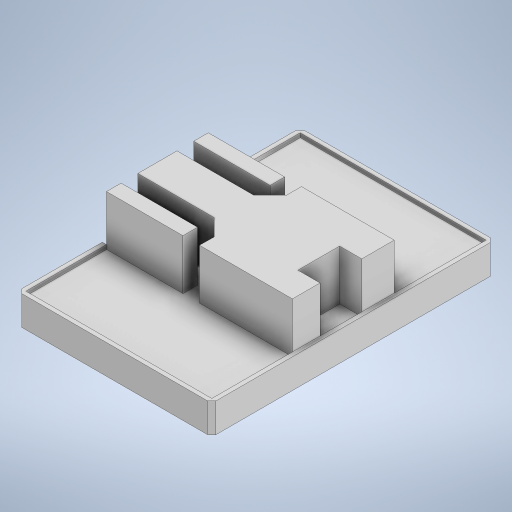
# Autodesk Inventor part: Suporte
Saved by Autodesk Inventor 2024 (Build 280153020, 153B)
## iProperties
Created: 2023-05-31
Part Number: Suporte
Material: Genérico
Document SubType Name: Modeling
Designer: victo
Density: 1 g/cm^3
Appearance: Padrão
Author: victo
Autodesk Inventor part; units mm, degrees
ref_plane "YZ Plane" through (0, 0, 0) normal (1, 0, 0) x (0, 1, 0)
ref_plane "XZ Plane" through (0, 0, 0) normal (0, 1, 0) x (-1, 0, 0)
ref_plane "XY Plane" through (0, 0, 0) normal (0, 0, 1) x (1, 0, 0)
sketch "Esboço1" plane through (0, 0, 0) normal (0, 1, 0) x (-1, 0, 0)
  line L0 (0.0003, 60.0007) -> (0.0003, 29.9998)
  line L1 (0.0003, 29.9998) -> (0.0003, 29.9999)
  line L2 (-0.9997, 29.9999) -> (-0.9997, 60.0007)
  line L3 (0.0003, 29.9999) -> (0.0003, 14.4635)
  line L4 (-0.9997, 14.4635) -> (-0.9997, 29.9999)
  line L5 (44.5003, 33.7635) -> (45.5003, 33.7635)
  line L6 (44.5003, 58.1254) -> (45.5003, 58.1254)
  line L7 (26.2003, 33.7635) -> (26.2003, 37.2635)
  line L8 (26.2003, 37.2635) -> (44.5003, 37.2635)
  line L9 (22.2003, 33.7635) -> (0.0003, 33.7635)
  line L10 (22.2003, 33.7635) -> (22.2003, 37.2635)
  line L11 (26.2003, 33.7635) -> (45.0003, 33.7635)
  line L12 (37.268, 41.2635) -> (44.5003, 41.2635)
  line L13 (22.2003, 37.2635) -> (26.2003, 41.2635)
  line L14 (37.268, 41.2635) -> (26.2003, 41.2635)
  line L15 (43.0622, 54.6254) -> (44.5003, 54.6254)
  line L16 (43.0622, 54.6254) -> (26.2003, 54.6254)
  line L17 (26.2003, 54.6254) -> (26.2003, 58.1254)
  line L18 (22.2003, 54.6254) -> (22.2503, 58.1254)
  line L19 (26.2003, 50.6254) -> (22.2003, 54.6254)
  line L20 (26.2003, 50.6254) -> (44.5003, 50.6254)
  line L21 (0.0003, 58.1254) -> (22.2503, 58.1254)
  line L22 (26.2003, 58.1254) -> (44.5003, 58.1254)
  line L23 (44.5003, 54.6254) -> (44.5003, 58.1254)
  line L24 (44.5003, 48.0257) -> (44.5003, 50.6254)
  line L25 (44.5003, 33.7635) -> (44.5003, 37.2635)
  line L26 (44.5003, 41.2635) -> (44.5003, 45.0257)
  line L27 (44.5003, 37.2635) -> (44.5003, 41.2635)
  line L28 (44.5003, 45.0257) -> (44.5003, 48.0257)
  line L29 (44.5003, 50.6254) -> (44.5003, 54.6254)
  line L30 (44.5003, 33.968) -> (44.5003, 11.768)
  line L31 (44.5003, 11.768) -> (0.0003, 11.768)
  line L32 (0.0003, 11.768) -> (0.0003, 14.4635)
  line L33 (45.5003, 33.7635) -> (45.5003, 11.768)
  line L34 (44.5003, 58.1254) -> (44.5003, 77.4254)
  line L35 (44.5003, 77.4254) -> (0.0003, 77.4254)
  line L36 (0.0003, 60.0007) -> (0.0003, 77.4254)
  line L37 (45.5003, 58.1254) -> (45.5003, 77.4254)
  line L38 (45.5003, 77.4254) -> (44.5003, 78.4254)
  line L39 (0.0003, 78.4254) -> (-0.9997, 77.4254)
  line L40 (0.0003, 78.4254) -> (44.5003, 78.4254)
  line L41 (-0.9997, 60.0007) -> (-0.9997, 77.4254)
  line L42 (0.0003, 10.768) -> (-0.9997, 11.768)
  line L43 (45.5003, 11.768) -> (44.5003, 10.768)
  line L44 (-0.9997, 11.768) -> (-0.9997, 14.4635)
  line L45 (0.0003, 10.768) -> (44.5003, 10.768)
  line L46 (4.3192, 41.5257) -> (5.3003, 41.5257)
  line L47 (4.8098, 51.5257) -> (5.3003, 51.5257)
  line L48 (5.3003, 41.5257) -> (5.3003, 51.5257)
  line L49 (4.3192, 41.5257) -> (0.0003, 41.5257)
  line L50 (4.8098, 51.5257) -> (0.0003, 51.5257)
  point P0 (0, 0)
  dimension "d40" = 1
  dimension "d86" = 44.5
  dimension "d90" = 1
  dimension "d91" = 1
  dimension "d94" = 4
  dimension "d116" = 22.2
  dimension "d118" = 19.3
  constraints: 102 end point, 22 perpendicular, 10 vertical, 9 point on line, 8 horizontal, 4 collinear, 2 parallel, 1 midpoint
  measures "d40" distance of L1.end L2.start
  measures "d86" distance of L21.start L6.start
  measures "d90" distance of L5.start L5.end
  measures "d91" distance of L6.start L6.end
  measures "d94" distance of L7.start L9.start
  measures "d116" distance of L30.start L30.end
  measures "d118" distance of L23.end L34.end
extrude "Extrusão30" add sketch "Esboço1" along normal blind 6 contours L36 L35 L34 L22 L17 L16 L15 L29 L20 L19 L18 L21 L0 | L50 L47 L48 L46 L49 L0 | L9 L10 L13 L14 L12 L27 L8 L7 L11 L30 L31 L32 L3 L0
extrude "Extrusão32" add sketch "Esboço1" along normal blind 18 contours L21 L18 L19 L20 L24 L28 L26 L12 L14 L13 L10 L9 L0 L49 L46 L48 L47 L50 | L23 L15 L16 L17 L22 | L11 L7 L8 L25
extrude "Extrusão33" add sketch "Esboço1" along normal blind 7 contours L0 L3 L32 L31 L30 L5 L33 L43 L45 L42 L44 L4 L2 L41 L39 L40 L38 L37 L6 L34 L35 L36
sketch "Esboço4" plane through (0, 0, 0) normal (0, -1, 0) x (1, 0, 0)
  line L0 (-44.5003, 11.768) -> (-0.0003, 11.768) projected
  line L1 (-0.0003, 77.4254) -> (-44.5003, 77.4254) projected
  line L2 (-44.5003, 33.7635) -> (-44.5003, 58.1254) projected
  line L3 (-0.0003, 41.5257) -> (-0.0003, 51.5257) projected
  circle A0 centre (-22.2503, 44.5969) radius 3.75
  line L4 (-26.2003, 58.1254) -> (-26.2003, 54.6254) projected
  line L5 (-22.2503, 58.1254) -> (-0.0003, 58.1254) projected
  arc A1 (-20.3067, 58.1254) -> (-24.2503, 58.5969) centre (-22.2503, 58.5969) ccw
  arc A2 (-24.2003, 30.597) -> (-20.2003, 30.597) centre (-22.2003, 30.597) ccw
  line L6 (-22.2003, 33.7635) -> (-0.0003, 33.7635) projected
  line L7 (-24.2003, 30.597) -> (-24.6441, 41.7103)
  line L8 (-20.2003, 30.597) -> (-19.853, 41.7132)
  line L9 (-24.2503, 58.5969) -> (-24.6458, 47.4821)
  line L10 (-20.2503, 58.5969) -> (-19.8549, 47.4821)
  point P0 (0, 0)
  point P1 (-20.2336, 58.1254)
  dimension "d141" = 7.5
  dimension "d155" = 4
  dimension "d156" = 4
  constraints: 9 end point, 9 point on circle, 3 centre point, 1 point on line
  measures "d141" diameter of A0
  measures "d155" diameter of A1
  measures "d156" diameter of A2
extrude "Extrusão35" cut sketch "Esboço4" against normal blind 3 contours A0 | A0 L9 A1 L5 L10 | L8 A2 L7 A0
